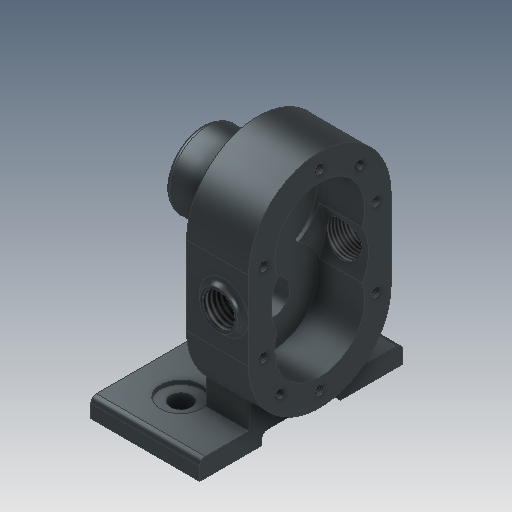
# Autodesk Inventor part: 泵体
Saved by Autodesk Inventor 2020 (Build 240168000, 168)
## iProperties
Created: 2021-04-21
Part Number: 泵体
Material: 铁，铸造
Document SubType Name: Modeling
Designer: Luorily
Density: 7.15 g/cm^3
Appearance: 灰口铁
Author: Luorily
Autodesk Inventor part; units mm, degrees
note: some values were not read from the file. Chosen so that the rebuilt part matches the saved one: direction of "孔8"; direction of "孔9".
ref_plane "YZ Plane" through (0, 0, 0) normal (1, 0, 0) x (0, 1, 0)
ref_plane "XZ Plane" through (0, 0, 0) normal (0, 1, 0) x (-1, 0, 0)
ref_plane "XY Plane" through (0, 0, 0) normal (0, 0, 1) x (1, 0, 0)
sketch "草图2" plane through (0, 0, 0) normal (0, 1, 0) x (-1, 0, 0)
  line L0 (29, 54) -> (-29, 54)
  line L1 (-29, 54) -> (-29, -54)
  line L2 (-29, -54) -> (29, -54)
  line L3 (29, -54) -> (29, 54)
  point P0 (0, 0)
  dimension "d2" = 58
  dimension "d3" = 108
  constraints: 8 end point, 2 parallel, 1 horizontal, 1 perpendicular
  measures "d2" distance of L2.end L1.end
  measures "d3" distance of L1.end L0.end
extrude "拉伸1" add sketch "草图2" against normal blind 10
sketch "草图3" plane through (0, -10, 0) normal (0, -1, 0) x (1, 0, 0)
  line L0 (29, -54) -> (29, 54) projected
  line L1 (-29, 54) -> (-29, -54) projected
  line L2 (29, 0) -> (29, -21)
  line L3 (29, -21) -> (-29, -21)
  line L4 (29, 0) -> (29, 21)
  line L5 (29, 21) -> (-29, 21)
  line L6 (-29, -21) -> (-29, 21)
  point P0 (0, 0)
  dimension "d6" = 21
  dimension "d7" = 21
  constraints: 10 end point, 4 point on line, 2 perpendicular, 1 collinear, 1 midpoint
  measures "d6" distance of L2.start L2.end
  measures "d7" distance of L2.start L4.end
extrude "拉伸2" cut sketch "草图3" against normal blind 6
sketch "草图4" plane through (0, 0, 0) normal (0, 1, 0) x (1, 0, 0)
  line L0 (29, -21) -> (29, -54) projected
  line L1 (29, -54) -> (-5, -54) construction
  line L2 (29, -54) -> (-29, -54) projected
  line L3 (-5, -54) -> (-5, -30) construction
  line L4 (-5, 54) -> (-5, 30) construction
  point P0 (0, 0)
  dimension "d10" = 34
  dimension "d11" = 24
  constraints: 6 end point, 2 coincident, 1 perpendicular, 1 point on line
  measures "d10" distance of L0.end L1.end
  measures "d11" distance of L1.end L3.end
hole "孔1" at (-5, 0, -30) at (-5, 0, 30) direction (0, -1, 0) diameter 11 depth 10 counterbore diameter 22 counterbore depth 2
sketch "草图5" plane through (0, 0, 0) normal (0, 1, 0) x (1, 0, 0)
  line L0 (29, -54) -> (29, 54) projected
  line L1 (29, -21) -> (29, 21) projected
  line L2 (29, 0) -> (29, -27.5)
  line L3 (29, -27.5) -> (6, -27.5)
  line L4 (6, -27.5) -> (6, 27.5)
  line L5 (6, 27.5) -> (29, 27.5)
  line L6 (29, 54) -> (29, 21) projected
  line L7 (29, 0) -> (29, 27.5)
  point P0 (0, 0)
  dimension "d21" = 27.5
  dimension "d23" = 23
  dimension "d24" = 55
  constraints: 10 end point, 2 perpendicular, 2 point on line, 1 collinear, 1 horizontal, 1 midpoint
  measures "d21" distance of L2.start L2.end
  measures "d23" distance of L2.end L3.end
  measures "d24" distance of L3.end L4.end
extrude "拉伸3" add sketch "草图5" along normal blind 20
sketch "草图6" plane through (29, -10, -54) normal (1, 0, 0) x (0, 0, -1)
  line L0 (-26.5, 10) -> (-26.5, 30) projected
  line L1 (-81.5, 30) -> (-26.5, 30) projected
  line L2 (-81.5, 10) -> (-81.5, 30) projected
  line L3 (-54, 10) -> (-54, 50) construction
  arc A0 (-92, 50) -> (-16, 50) centre (-54, 50) ccw
  line L4 (-54, 50) -> (-54, 92) construction
  arc A1 (-16, 92) -> (-92, 92) centre (-54, 92) ccw
  line L5 (-16, 50) -> (-16, 92)
  line L6 (-92, 50) -> (-92, 92)
  point P0 (-81.5, 23.775)
  point P1 (-26.5, 23.775)
  dimension "d27" = 40
  dimension "d28" = 76
  dimension "d29" = 42
  dimension "d30" = 76
  constraints: 8 end point, 4 point on circle, 3 vertical, 2 centre point, 2 coincident, 1 parallel
  measures "d27" distance of L3.start L3.end
  measures "d28" diameter of A0
  measures "d29" distance of L4.start L4.end
  measures "d30" diameter of A1
extrude "拉伸4" add sketch "草图6" along normal blind 10 and the other way blind 23
sketch "草图7" plane through (39, -10, -54) normal (1, 0, 0) x (0, 0, -1)
  arc A0 (-92, 50) -> (-16, 50) centre (-54, 50) ccw projected
  arc A1 (-16, 92) -> (-92, 92) centre (-54, 92) ccw projected
  point P0 (-54, 10)
  constraints: 2 coincident
hole "孔2" at (39, 82, 0) at (39, 40, 0) direction (-1, 0, 0) diameter 48 depth 25
sketch "草图8" plane through (39, -10, -54) normal (1, 0, 0) x (0, 0, -1)
  line L0 (-42.381, 71) -> (-65.619, 71)
  point P0 (-54, 10)
  point P1 (-54, 71)
  constraints: 2 end point, 1 horizontal, 1 midpoint
hole "孔3" at (39, 61, 0) direction (-1, 0, 0) diameter 52 depth 23
sketch "草图9" plane through (6, 0, -27.5) normal (-1, 0, 0) x (0, 0, 1)
  arc A0 (-10.5, 40) -> (0, 13.775) centre (27.5, 40) ccw projected
  circle A1 centre (27.5, 40) radius 15
  point P0 (27.5, 0)
  dimension "d49" = 30
  constraints: 1 centre point, 1 coincident
  measures "d49" diameter of A1
extrude "拉伸5" add sketch "草图9" along normal blind 18
sketch "草图11" plane through (6, 0, -27.5) normal (-1, 0, 0) x (0, 0, 1)
  arc A0 (65.5, 82) -> (-10.5, 82) centre (27.5, 82) ccw projected
  circle A1 centre (27.5, 82) radius 20
  point P0 (27.5, 0)
  dimension "d59" = 40
  constraints: 1 centre point, 1 coincident
  measures "d59" diameter of A1
extrude "拉伸6" add sketch "草图11" along normal blind 30
sketch "草图12" plane through (14, 82, 0) normal (1, 0, 0) x (0, 0, -1)
  arc A0 (11.619, -21) -> (-11.619, -21) centre (0, 0) ccw projected
  point P0 (0, -42)
  point P1 (0, -82)
  constraints: 1 coincident
sketch "草图15" plane through (-24, 82, 0) normal (-1, 0, 0) x (0, 0, 1)
  circle A0 centre (0, 0) radius 20 projected
  point P0 (0, -82)
  constraints: 1 coincident
hole "孔5" at (-24, 82, 0) direction (1, 0, 0) diameter 23.752 depth 67.1 thread size "M27x3" designation "M27" class "6H" standard "GB Metric profile"
hole "孔6" at (14, 40, 0) direction (-1, 0, 0) diameter 18 depth 20 tip angle 118
sketch "草图16" plane through (39, 82, -38) normal (0, 0, -1) x (-1, 0, 0)
  circle A0 centre (13, -21) radius 10
  line L0 (0, -42) -> (0, 0) projected
  line L1 (0, -21) -> (13, -21)
  point P0 (39, -82)
  dimension "d78" = 20
  dimension "d99" = 13
  constraints: 2 end point, 1 centre point, 1 horizontal, 1 midpoint
  measures "d78" diameter of A0
  measures "d99" distance of L1.start L1.end
extrude "拉伸7" add sketch "草图16" along normal blind 3
sketch "草图17" plane through (6, 40, 38) normal (0, 0, 1) x (1, 0, 0)
  line L0 (33, 0) -> (33, 42) projected
  line L1 (33, 21) -> (20, 21)
  circle A0 centre (20, 21) radius 10
  point P0 (-6, -40)
  dimension "d81" = 13
  dimension "d82" = 20
  constraints: 2 end point, 1 centre point, 1 coincident, 1 horizontal, 1 midpoint
  measures "d81" distance of L1.start L1.end
  measures "d82" diameter of A0
extrude "拉伸8" add sketch "草图17" along normal blind 3
sketch "草图18" plane through (26, 61, 41) normal (0, 0, 1) x (1, 0, 0)
  circle A0 centre (0, 0) radius 10 projected
  point P0 (-26, -61)
  constraints: 1 coincident
hole "孔8" at (26, 61, 41) direction (0, 0, -1) diameter 17.294 end up to surface thread size "M20x2.5" designation "M20" class "6H" standard "GB Metric profile"
sketch "草图20" plane through (26, 61, -41) normal (0, 0, -1) x (-1, 0, 0)
  circle A0 centre (0, 0) radius 10 projected
  point P0 (26, -61)
  constraints: 1 coincident
hole "孔9" at (26, 61, -41) direction (0, 0, 1) diameter 18.631 end up to surface thread size "G20.955x1.814" designation "G 1/2" standard "GB Pipe Threads without seal"
sketch "草图21" plane through (39, -10, -54) normal (1, 0, 0) x (0, 0, -1)
  arc A0 (-76.585, 58.119) -> (-31.415, 58.119) centre (-54, 50) ccw projected
  arc A1 (-16, 92) -> (-92, 92) centre (-54, 92) ccw projected
  circle A2 centre (-54, 50) radius 30
  circle A3 centre (-54, 92) radius 30
  point P0 (-54, 10)
  point P1 (-84, 92)
  point P2 (-24, 92)
  point P3 (-54, 122)
  point P4 (-54, 20)
  point P5 (-24, 50)
  point P6 (-84, 50)
  dimension "d107" = 60
  dimension "d108" = 60
  constraints: 6 point on circle, 2 centre point, 2 coincident
  measures "d107" diameter of A2
  measures "d108" diameter of A3
hole "孔10" at (39, 82, 30) at (39, 82, -30) at (39, 112, 0) at (39, 10, 0) at (39, 40, -30) at (39, 40, 30) direction (-1, 0, 0) diameter 4.917 depth 15 tip angle 118 thread size "M6x1" designation "M6" class "6H" standard "GB Metric profile"
sketch "草图22" plane through (39, -10, -54) normal (1, 0, 0) x (0, 0, -1)
  arc A0 (-31.415, 83.881) -> (-76.585, 83.881) centre (-54, 92) ccw projected
  arc A1 (-76.585, 58.119) -> (-31.415, 58.119) centre (-54, 50) ccw projected
  line L0 (-54, 50) -> (-16, 50) construction
  line L1 (-54, 92) -> (-32.7868, 113.2132)
  line L2 (-54, 92) -> (-24, 92) construction
  line L3 (-54, 50) -> (-75.2132, 28.7868)
  line L4 (-54, 50) -> (-24, 50) construction
  point P0 (-54, 10)
  dimension "d117" = 30
  dimension "d118" = 45
  dimension "d119" = 30
  dimension "d120" = 135
  constraints: 10 end point, 3 horizontal, 2 coincident, 2 equal length
  measures "d117" distance of L1.start L1.end
  measures "d118" angle of L2 L1
  measures "d119" distance of L0.start L3.end
  measures "d120" angle of L3 L4
hole "孔11" at (39, 103.2132, -21.2132) at (39, 18.7868, 21.2132) direction (-1, 0, 0) diameter 5 depth 8 tip angle 118
sketch "草图23" plane through (6, 0, -27.5) normal (-1, 0, 0) x (0, 0, 1)
  circle A0 centre (27.5, 82) radius 20 projected
  circle A1 centre (27.5, 40) radius 15 projected
  line L0 (55, 0) -> (0, 0) projected
  line L1 (27.5, 0) -> (32.5, 0)
  line L2 (32.5, 0) -> (32.5, 62.6351)
  line L3 (27.5, 0) -> (22.5, 0)
  line L4 (22.5, 0) -> (22.5, 62.6351)
  point P0 (22.5, 25.8579)
  point P1 (32.5, 25.8579)
  point P2 (22.5, 54.1421)
  point P3 (32.5, 54.1421)
  dimension "d128" = 5
  dimension "d129" = 5
  constraints: 8 end point, 2 perpendicular, 2 point on line, 2 other
  measures "d128" distance of L1.start L1.end
  measures "d129" distance of L1.start L3.end
extrude "拉伸9" add sketch "草图23" along normal blind 14 contours A0 L2 A1 L4 | A1 L2 L0 L4
fillet "圆角1" radius 3 11 edges at (0, 0, -54) (0, 0, 54) (-8, 0, 0) (-1, 0, -5) (-1, 0, 5) (0, -4, -21) (0, -4, 21) (16, 61, 38) (36, 61, -38) (-1, 62.6351, 5) (-1, 62.6351, -5)
fillet "圆角2" radius 3 2 edges at (-12, 40, -15) (-24, 82, -20)
